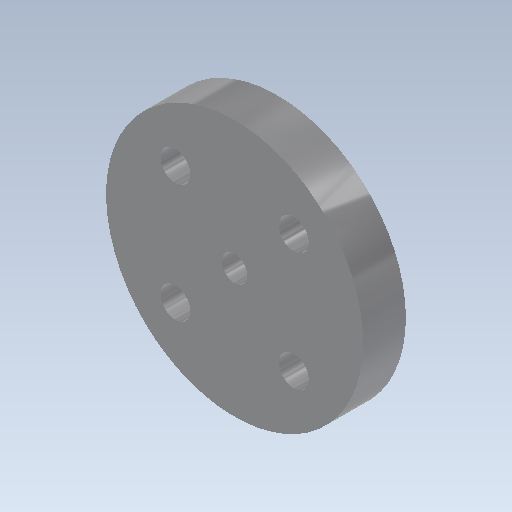
# Autodesk Inventor part: encoder_spacer
Saved by Autodesk Inventor 2020 (Build 240168000, 168)
## iProperties
Created: 2016-11-14
Part Number: encoder_spacer
Material: Generic
Document SubType Name: Sheet Metal
Designer: jous
Density: 1 g/cm^3
Appearance: Default
Sheet Metal Rule: Default
Mass: 3.30595 g
Surface Area: 20.6098 cm^2
Volume: 3.30595 cm^3
Author: jous
Autodesk Inventor part; units mm, degrees
ref_plane "YZ Plane" through (0, 0, 0) normal (1, 0, 0) x (0, 1, 0)
ref_plane "XZ Plane" through (0, 0, 0) normal (0, 1, 0) x (-1, 0, 0)
ref_plane "XY Plane" through (0, 0, 0) normal (0, 0, 1) x (1, 0, 0)
sketch "Sketch1" plane through (0, 0, 0) normal (0, 0, 1) x (1, 0, 0)
  circle A0 centre (0, 0) radius 15
  line L0 (-73.4722, 0) -> (96.5278, 0) construction
  line L1 (0, 0) -> (0, 31) construction
  circle A1 centre (0, 0) radius 1.5
  circle A2 centre (-6.9148, 6.9148) radius 1.7526
  line L2 (0, 0) -> (-14.5685, 14.5685) construction
  circle A3 centre (-6.9148, -6.9148) radius 1.7526
  circle A4 centre (6.9148, -6.9148) radius 1.7526
  circle A5 centre (6.9148, 6.9148) radius 1.7526
  point P0 (0, 0)
  dimension "d4" = 30
  dimension "d10" = 3
  dimension "d11" = 3.5052
  dimension "d12" = 45
  dimension "d13" = 6.9148
  dimension "d16" = 360
  constraints: 6 centre point, 6 end point, 2 coincident, 2 point on line, 1 perpendicular, 9 other
  measures "d4" diameter of A0
  measures "d10" diameter of A1
  measures "d11" diameter of A2
  measures "d12" angle of L0 L2
  measures "d13" distance from line of L0 A2.centre
extrude "Extrusion1" add sketch "Sketch1" along normal blind 5 contours A0 | A1 | A2 | A3 | A4 | A5
extrude "Extrusion2" cut sketch "Sketch1" along normal through all contours A1 | A2 | A3 | A4 | A5
equation "\"BendRadius\" = Thickness"
equation "\"BendReliefWidth\" = Thickness"
equation "\"BendReliefDepth\" = 0.5 * Thickness"
equation "\"CornerReliefSize\" = 4 * Thickness"
equation "\"MinimumRemnant\" = 2 * Thickness"
equation "\"TransitionRadius\" = BendRadius"
equation "\"JacobiRadiusSize\" = Thickness"
equation "\"GapSize\" = Thickness"
equation "\"Thickness\" = 0.5"
body "Solid1"
